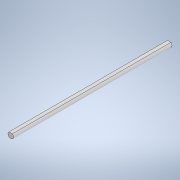
# Autodesk Inventor part: Eje_Engranes_llanta
Saved by Autodesk Inventor 2021 (Build 250183000, 183)
## iProperties
Created: 2021-02-06
Part Number: Eje_Engranes_llanta
Material: Genérico
Document SubType Name: Modeling
Designer: rotje
Density: 1 g/cm^3
Appearance: Valor por defecto
Author: rotje
Autodesk Inventor part; units mm, degrees
ref_plane "YZ Plane" through (0, 0, 0) normal (1, 0, 0) x (0, 1, 0)
ref_plane "XZ Plane" through (0, 0, 0) normal (0, 1, 0) x (-1, 0, 0)
ref_plane "XY Plane" through (0, 0, 0) normal (0, 0, 1) x (1, 0, 0)
sketch "Boceto1" plane through (0, 0, 0) normal (0, 0, 1) x (1, 0, 0)
  circle A0 centre (0, 0) radius 7.5
  dimension "d0" = 15
  constraints: 1 centre point, 1 coincident
  measures "d0" diameter of A0
extrude "Extrusión1" add sketch "Boceto1" along normal mid plane 420
sketch "Boceto2" plane through (0, 0, 210) normal (0, 0, 1) x (1, 0, 0)
  circle A0 centre (0, 0) radius 7.5 projected
  line L0 (0, 0) -> (0, 6)
  line L1 (0, 6) -> (-4.5, 6)
  line L2 (0, 6) -> (4.5, 6)
  arc A1 (4.5, 6) -> (-4.5, 6) centre (0, 0) ccw
  dimension "d3" = 6
  constraints: 6 end point, 4 point on circle, 1 centre point, 1 concentric, 1 horizontal, 1 point on line, 1 vertical
  measures "d3" distance of L0.start L0.end
extrude "Extrusión2" cut sketch "Boceto2" against normal blind 420 contours L2 L1 A0 picked at (-2.5399, 6.2735)
